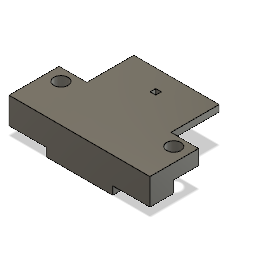
Testing_Stage (Autodesk Fusion 360 archive; units mm, degrees)
design "sensor slit"
Autodesk Fusion 360 part; units mm, degrees
sketch "board contact" plane through (0, 0, 0) normal (0, 1, 0) x (1, 0, 0)
  line L0 (12.7, -1.75) -> (-12.7, -1.75)
  line L1 (-12.7, -1.75) -> (-12.7, 1.75)
  line L2 (-12.7, 1.75) -> (12.7, 1.75)
  line L3 (12.7, 1.75) -> (12.7, -1.75)
  line L4 (61.7395, 0) -> (-97.655, 0) construction
  line L5 (0, -60.5274) -> (0, 48.7233) construction
  line L6 (8.2, 2.75) -> (12.7, 2.75)
  line L7 (12.7, 2.75) -> (12.7, 1.75)
  line L8 (12.7, 1.75) -> (8.2, 1.75)
  line L9 (8.2, 1.75) -> (8.2, 2.75)
  line L10 (-12.7, 3) -> (2.45, 3)
  line L11 (2.45, 3) -> (2.45, 1.75)
  line L12 (2.45, 1.75) -> (-12.7, 1.75)
  line L13 (-12.7, 1.75) -> (-12.7, 3)
  circle A0 centre (10.16, 0.79) radius 1.27
  circle A1 centre (-10.16, 0.79) radius 1.27
  line L14 (-10.16, 0.79) -> (10.16, 0.79) construction
  line L15 (2.45, 9.25) -> (-1.95, 9.25)
  line L16 (-1.95, 9.25) -> (-1.95, 3)
  line L17 (-1.95, 3) -> (2.45, 3)
  line L18 (2.45, 3) -> (2.45, 9.25)
  line L19 (0.5, 7.19) -> (-0.5, 7.19)
  line L20 (-0.5, 7.19) -> (-0.5, 8.19)
  line L21 (-0.5, 8.19) -> (0.5, 8.19)
  line L22 (0.5, 8.19) -> (0.5, 7.19)
  line L23 (7.7, 11.45) -> (-7.7, 11.45)
  line L24 (-7.7, 11.45) -> (-7.7, -1.75)
  line L25 (-7.7, -1.75) -> (7.7, -1.75)
  line L26 (7.7, -1.75) -> (7.7, 11.45)
  line L27 (8.2, 2.75) -> (7.7, 2.75)
  line L28 (-0.5, 7.69) -> (0.5, 7.69) construction
  dimension "d1" = 3.5
  dimension "d2" = 25.4
  dimension "d3" = 4.5
  dimension "d4" = 4.5
  dimension "d7" = 4.75
  dimension "d10" = 20.32
  dimension "d11" = 2.54
  dimension "d12" = 2.54
  dimension "d13" = 10.25
  dimension "d14" = 10.75
  dimension "d15" = 11
  dimension "d17" = 1
  dimension "d18" = 1
  dimension "d20" = 5
  dimension "d21" = 5
  dimension "d22" = 13.2
  dimension "d39" = 9.44
  constraint horizontal L0
  constraint vertical L1
  constraint horizontal L2
  constraint vertical L3
  constraint perpendicular L3 L4
  constraint vertical L5
  constraint coincident origin L5
  constraint coincident origin L4
  constraint symmetric L1 L3 L5
  constraint symmetric L0 L2 L4
  constraint horizontal L6
  constraint vertical L7
  constraint horizontal L8
  constraint vertical L9
  constraint collinear L3 L7
  constraint collinear L2 L8
  constraint horizontal L10
  constraint vertical L11
  constraint horizontal L12
  constraint vertical L13
  constraint collinear L1 L13
  constraint collinear L2 L12
  constraint equal A0 A1
  constraint coincident A1.centre L14.start
  constraint coincident A0.centre L14.end
  constraint horizontal L14
  constraint symmetric L5 A0.centre A1.centre
  constraint horizontal L15
  constraint vertical L16
  constraint horizontal L17
  constraint vertical L18
  constraint collinear L10 L17
  constraint collinear L11 L18
  constraint horizontal L19
  constraint vertical L20
  constraint horizontal L21
  constraint vertical L22
  constraint symmetric L5 L20 L22
  constraint horizontal L23
  constraint vertical L24
  constraint horizontal L25
  constraint vertical L26
  constraint collinear L0 L25
  constraint coincident L26 L27.end
  constraint perpendicular L26 L27
  constraint midpoint L20 L28.start
  constraint midpoint L22 L28.end
  measures "d1" distance of L0.end L1.end
  measures "d2" distance of L0.start L0.end
  measures "d3" distance of L0 L6
  measures "d4" distance of L6.start L6.end
  measures "d7" distance of L0 L10
  measures "d10" distance of A0.centre A1.centre
  measures "d11" distance of L0 A0.centre
  measures "d12" diameter of A0
  measures "d13" distance of L3 L18
  measures "d14" distance of L1 L16
  measures "d15" distance of L0 L15
  measures "d17" distance of L19.start L19.end
  measures "d18" distance of L19.end L20.end
  measures "d20" distance of L3 L26
  measures "d21" distance of L13 L24
  measures "d22" distance of L0 L23
  measures "d39" distance of L0 L28
extrude "Extrude1" add sketch "board contact" along normal blind 3.2 contours L0 L2 L3 L8 A0 L26 | L0 L2 L12 L24 L25 L26 | L2 L6 L7 L8 L9 A0 | L0 L1 L2 L12 A1 L24 | L2 L9 L26 L27 | L2 L10 L11 L15 L16 L18 L23 L24 L26 | L2 L10 L11 L12 L17 L24 | L2 L10 L12 L13 A1 L24 | L10 L15 L16 L17 L18
extrude "Extrude2" cut sketch "board contact" along normal blind 2 contours L2 L9 L26 L27 | L2 L10 L11 L15 L16 L18 L23 L24 L26 | L2 L10 L11 L12 L17 L24 | L10 L15 L16 L17 L18
sketch "vertical extension" plane through (0, 0, 0) normal (0, -1, 0) x (1, 0, 0)
  line L0 (-12.7, -3) -> (-7.7, -3)
  line L1 (-7.7, -1.75) -> (8.2, -1.75)
  line L2 (8.2, -1.75) -> (8.2, -2.75)
  line L3 (8.2, -2.75) -> (12.7, -2.75)
  line L4 (12.7, -2.75) -> (12.7, 1.75)
  line L5 (12.7, 1.75) -> (-12.7, 1.75)
  line L6 (-12.7, 1.75) -> (-12.7, -3)
  circle A0 centre (10.16, -0.79) radius 1.27
  circle A1 centre (-10.16, -0.79) radius 1.27
  line L7 (-6, 6.05) -> (6, 6.05)
  line L8 (6, 6.05) -> (6, 4.55)
  line L9 (6, 4.55) -> (-6, 4.55)
  line L10 (-6, 4.55) -> (-6, 6.05)
  line L11 (0, 1.75) -> (0, -6.45) construction
  line L12 (-12.7, 6.05) -> (12.7, 6.05)
  line L13 (12.7, 6.05) -> (12.7, 1.75)
  line L14 (12.7, 1.75) -> (-12.7, 1.75)
  line L15 (-12.7, 1.75) -> (-12.7, 6.05)
  line L16 (-7.7, -3) -> (-7.7, -1.75)
  dimension "d25" = 12
  dimension "d26" = 1.5
  dimension "d29" = 4.3
  constraint horizontal L7
  constraint vertical L8
  constraint horizontal L9
  constraint vertical L10
  constraint midpoint L5 L11.start
  constraint perpendicular L5 L11
  constraint symmetric L8 L10 L11
  constraint horizontal L12
  constraint vertical L13
  constraint horizontal L14
  constraint vertical L15
  constraint collinear L4 L13
  constraint collinear L6 L15
  constraint collinear L7 L12
  constraint collinear L5 L14
  measures "d25" distance of L7.start L7.end
  measures "d26" distance of L7.end L8.end
  measures "d29" distance of L12.start L5.end
extrude "Extrude4" add sketch "vertical extension" along normal blind -3.2 and the other way blind -1.6 contours L5 L8 L9 L10 L12 L13 L14 L15 | L7 L8 L9 L10 L12
extrude "Extrude3" add sketch "vertical extension" along normal blind 3.1 contours L7 L8 L9 L10 L12
extrude "Extrude6" cut 1 faces at (-2.5667, 0, -0.6331) along direction (0, 1, 0) blind 0.5

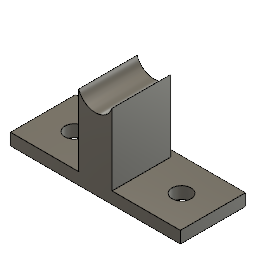
design "led cover"
Autodesk Fusion 360 part; units mm, degrees
sketch "Sketch1" plane through (0, 0, 0) normal (0, 1, 0) x (1, 0, 0)
  line L0 (2.5, -4.375) -> (-2.5, -4.375)
  line L1 (-2.5, -4.375) -> (-2.5, 4.375)
  line L2 (-2.5, 4.375) -> (2.5, 4.375)
  line L3 (2.5, 4.375) -> (2.5, -4.375)
  line L4 (0, -17.6215) -> (0, 10.113) construction
  line L5 (14.6118, 0) -> (-14.9327, 0) construction
  dimension "d1" = 5
  dimension "d2" = 8.75
  constraint horizontal L0
  constraint vertical L1
  constraint horizontal L2
  constraint vertical L3
  constraint parallel L1 L4
  constraint perpendicular L3 L5
  constraint coincident origin L5
  constraint coincident origin L4
  constraint symmetric L1 L3 L4
  constraint symmetric L0 L2 L5
  measures "d1" distance of L0.start L0.end
  measures "d2" distance of L0.end L1.end
extrude "Extrude1" add sketch "Sketch1" along normal blind 8.875
sketch "Sketch2" plane through (0, 0, 4.375) normal (0, 0, 1) x (1, 0, 0)
  line L0 (-2.5, 0) -> (2.5, 0)
  line L1 (2.5, 0) -> (2.5, 8.875)
  line L2 (2.5, 8.875) -> (-2.5, 8.875)
  line L3 (-2.5, 8.875) -> (-2.5, 0)
  line L4 (-2.5, 8.875) -> (2.5, 8.875)
  line L5 (2.5, 8.875) -> (2.5, 11.5)
  line L6 (2.5, 11.5) -> (-2.5, 11.5)
  line L7 (-2.5, 11.5) -> (-2.5, 8.875)
  circle A0 centre (0, 11.5) radius 2.625
  line L8 (0, 0) -> (0, 8.875) construction
  dimension "d10" = 5.25
  constraint horizontal L4
  constraint vertical L5
  constraint horizontal L6
  constraint vertical L7
  constraint coincident L2.end L3.start
  constraint tangent L4 A0
  constraint coincident L8.start origin
  constraint midpoint L4 L8.end
  constraint perpendicular L4 L8
  constraint coincident A0.centre L8
  constraint coincident L6 A0.centre
  measures "d10" diameter of A0
extrude "Extrude3" add sketch "Sketch2" against normal blind 8.75 contours L2 L4 L7 A0 | L2 L4 L5 A0
sketch "Sketch3" plane through (0, 0, 0) normal (0, -1, 0) x (1, 0, 0)
  line L0 (-2.5, -4.375) -> (2.5, -4.375)
  line L1 (2.5, -4.375) -> (2.5, 4.375)
  line L2 (2.5, 4.375) -> (-2.5, 4.375)
  line L3 (-2.5, 4.375) -> (-2.5, -4.375)
  line L4 (-12.7, 4.375) -> (12.7, 4.375)
  line L5 (12.7, 4.375) -> (12.7, -5.375)
  line L6 (12.7, -5.375) -> (-12.7, -5.375)
  line L7 (-12.7, -5.375) -> (-12.7, 4.375)
  line L8 (0, 4.375) -> (0, -4.375) construction
  line L9 (12.7, -0.5) -> (-12.7, -0.5) construction
  circle A0 centre (-8, -0.5) radius 1.42
  circle A1 centre (8, -0.5) radius 1.42
  dimension "d16" = 25.4
  dimension "d17" = 2.84
  dimension "d18" = 16
  dimension "d21" = 9.75
  dimension "d22" = 4.875
  constraint horizontal L4
  constraint vertical L5
  constraint horizontal L6
  constraint vertical L7
  constraint midpoint L2 L8.start
  constraint midpoint L0 L8.end
  constraint midpoint L4 L8.start
  constraint coincident L9 A0.centre
  constraint coincident L9 A1.centre
  constraint equal A0 A1
  constraint symmetric L8 A0 A1
  measures "d16" distance of L4.start L4.end
  measures "d17" diameter of A0
  measures "d18" distance of A0.centre A1.centre
  measures "d21" distance of L4.start L6.end
  measures "d22" distance of L4 L9
extrude "Extrude5" add sketch "Sketch3" along normal blind 1.8
